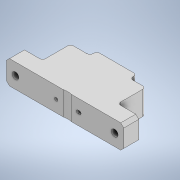
# Autodesk Inventor part: ADAPTER_new-focus-8821
Saved by Autodesk Inventor 2020 (Build 240168000, 168)
## iProperties
Created: 2021-08-06
Part Number: ADAPTER_new-focus-8821
Material: Generic
Document SubType Name: Modeling
Designer: paige
Density: 1 g/cm^3
Appearance: Default
Author: paige
Autodesk Inventor part; units mm, degrees
ref_plane "YZ Plane" through (0, 0, 0) normal (1, 0, 0) x (0, 1, 0)
ref_plane "XZ Plane" through (0, 0, 0) normal (0, 1, 0) x (-1, 0, 0)
ref_plane "XY Plane" through (0, 0, 0) normal (0, 0, 1) x (1, 0, 0)
sketch "Sketch1" plane through (0, 0, 0) normal (0, 0, 1) x (1, 0, 0)
  line L0 (-38.9875, 7.874) -> (38.9875, 7.874)
  line L1 (38.9875, 7.874) -> (38.9875, -7.874)
  line L2 (38.9875, -7.874) -> (-38.9875, -7.874)
  line L3 (-38.9875, -7.874) -> (-38.9875, 7.874)
  point P0 (0, 0)
  dimension "d2" = 77.975
  dimension "d3" = 38.9875
  dimension "d6" = 15.748
  dimension "d7" = 7.874
  constraints: 8 end point, 2 parallel, 1 horizontal, 1 perpendicular
  measures "d2" distance of L0.start L0.end
  measures "d3" distance from line of L1 point (0, 0)
  measures "d6" distance of L2.end L0.start
  measures "d7" distance from line of L2 point (0, 0)
extrude "Extrusion1" add sketch "Sketch1" along normal blind 33.1075
sketch "Sketch2" plane through (0, 0, 0) normal (0, 0, -1) x (-1, 0, 0)
  line L0 (38.9875, 7.874) -> (38.9875, -7.874) projected
  line L1 (-38.9875, -7.874) -> (-38.9875, 7.874) projected
  line L2 (38.9875, -7.874) -> (-38.9875, -7.874) projected
  line L3 (-38.9875, 7.874) -> (38.9875, 7.874) projected
  line L4 (38.9875, -7.874) -> (26.9875, -7.874)
  line L5 (26.9875, -7.874) -> (26.9875, 7.874)
  line L6 (26.9875, 7.874) -> (38.9875, 7.874)
  line L7 (38.9875, 7.874) -> (38.9875, -7.874)
  line L8 (-38.9875, -7.874) -> (-26.9875, -7.874)
  line L9 (-26.9875, -7.874) -> (-26.9875, 7.874)
  line L10 (-26.9875, 7.874) -> (-38.9875, 7.874)
  line L11 (-38.9875, 7.874) -> (-38.9875, -7.874)
  line L12 (38.9875, -7.874) -> (-38.9875, -7.874) projected
  line L13 (12.0525, -7.874) -> (-14.5415, -7.874)
  line L14 (-14.5415, -7.874) -> (-14.5415, 7.874)
  line L15 (-14.5415, 7.874) -> (12.0525, 7.874)
  line L16 (12.0525, 7.874) -> (12.0525, -7.874)
  line L17 (26.9875, -7.874) -> (12.0525, -7.874)
  line L18 (12.0525, -7.874) -> (12.0525, 7.874)
  line L19 (12.0525, 7.874) -> (26.9875, 7.874)
  line L20 (26.9875, 7.874) -> (26.9875, -7.874)
  line L21 (-14.5415, -7.874) -> (-26.9875, -7.874)
  line L22 (-26.9875, -7.874) -> (-26.9875, 7.874)
  line L23 (-26.9875, 7.874) -> (-14.5415, 7.874)
  line L24 (-14.5415, 7.874) -> (-14.5415, -7.874)
  line L25 (26.9875, -7.874) -> (24.9875, -7.874)
  line L26 (24.9875, -7.874) -> (24.9875, 7.874)
  line L27 (24.9875, 7.874) -> (26.9875, 7.874)
  line L28 (26.9875, 7.874) -> (26.9875, -7.874)
  line L29 (-26.9875, -7.874) -> (-24.9875, -7.874)
  line L30 (-24.9875, -7.874) -> (-24.9875, 7.874)
  line L31 (-24.9875, 7.874) -> (-26.9875, 7.874)
  line L32 (-26.9875, 7.874) -> (-26.9875, -7.874)
  point P0 (0, 0)
  point P1 (38.9875, 0)
  point P2 (-38.9875, 0)
  point P3 (-1.5875, 0)
  point P4 (32.9875, 0)
  point P5 (-32.9875, 0)
  point P6 (-14.5415, -7.874)
  point P7 (-24.9875, 7.874)
  point P8 (24.9875, 7.874)
  dimension "d4" = 0
  dimension "d5" = 0
  dimension "d8" = 12
  dimension "d9" = 12
  dimension "d14" = 6
  dimension "d15" = 15.748
  dimension "d16" = 7.874
  dimension "d17" = 6
  dimension "d18" = 7.874
  dimension "d19" = 12.954
  dimension "d20" = 13.64
  dimension "d72" = 25.4
  dimension "d74" = 7.874
  dimension "d83" = 2
  dimension "d84" = 2
  constraints: 56 end point, 14 parallel, 7 horizontal, 7 perpendicular, 6 point on line, 2 midpoint
  measures "d4" vertical distance of point (38.987, 0) point (0, 0)
  measures "d5" vertical distance of point (0, 0) point (-38.987, 0)
  measures "d8" distance between parallel lines of L5 L0
  measures "d9" distance between parallel lines of L1 L9
  measures "d14" distance from line of L5 point (32.987, 0)
  measures "d15" distance of L0.start L0.end
  measures "d16" distance from line of L2 point (32.987, 0)
  measures "d17" distance from line of L9 point (-32.987, 0)
  measures "d18" distance from line of L2 point (-32.987, 0)
  measures "d19" distance from line of L14 point (-1.587, 0)
  measures "d20" distance from line of L16 point (-1.587, 0)
  measures "d72" distance from line of L22 point (-1.587, 0)
  measures "d74" distance from line of L12 point (-1.587, 0)
  measures "d83" distance between parallel lines of L26 L20
  measures "d84" distance between parallel lines of L30 L9
hole "Hole1" at (-32.9875, 0, 0) at (32.9875, 0, 0) direction (0, 0, 1) diameter 4.5 end through all counterbore diameter 8 counterbore depth 30.11 clearance for "Socket Head Cap Screw" size "#8" standard "Ansi Unified Screw Threads"
sketch "Sketch4" plane through (0, 0, 33.1075) normal (0, 0, 1) x (1, 0, 0)
  line L0 (38.9875, 7.874) -> (38.9875, -7.874)
  line L1 (-38.9875, -7.874) -> (-38.9875, 7.874)
  line L2 (38.9875, -7.874) -> (-38.9875, -7.874)
  line L3 (-38.9875, 7.874) -> (38.9875, 7.874)
  line L4 (38.9875, -7.874) -> (26.9875, -7.874)
  line L5 (26.9875, -7.874) -> (26.9875, 7.874)
  line L6 (26.9875, 7.874) -> (38.9875, 7.874)
  line L7 (38.9875, 7.874) -> (38.9875, -7.874)
  line L8 (-38.9875, -7.874) -> (-26.9875, -7.874)
  line L9 (-26.9875, -7.874) -> (-26.9875, 7.874)
  line L10 (-26.9875, 7.874) -> (-38.9875, 7.874)
  line L11 (-38.9875, 7.874) -> (-38.9875, -7.874)
  line L12 (38.9875, -7.874) -> (-38.9875, -7.874)
  line L13 (14.5415, -7.874) -> (-12.0525, -7.874)
  line L14 (-12.0525, -7.874) -> (-12.0525, 7.874)
  line L15 (-12.0525, 7.874) -> (14.5415, 7.874)
  line L16 (14.5415, 7.874) -> (14.5415, -7.874)
  line L17 (26.9875, -7.874) -> (14.5415, -7.874)
  line L18 (14.5415, -7.874) -> (14.5415, 7.874)
  line L19 (14.5415, 7.874) -> (26.9875, 7.874)
  line L20 (26.9875, 7.874) -> (26.9875, -7.874)
  line L21 (-12.0525, -7.874) -> (-26.9875, -7.874)
  line L22 (-26.9875, -7.874) -> (-26.9875, 7.874)
  line L23 (-26.9875, 7.874) -> (-12.0525, 7.874)
  line L24 (-12.0525, 7.874) -> (-12.0525, -7.874)
  point P0 (0, 0)
  point P1 (0, 0)
  point P2 (0, 0)
  point P3 (38.9875, 0)
  point P4 (-38.9875, 0)
  point P5 (1.5875, 0.076)
  point P6 (32.9875, 0)
  point P7 (-32.9875, 0)
  dimension "d48" = 0
  dimension "d49" = 0
  dimension "d50" = 12
  dimension "d51" = 12
  dimension "d54" = 6
  dimension "d55" = 15.748
  dimension "d56" = 7.874
  dimension "d57" = 6
  dimension "d58" = 7.874
  dimension "d59" = 13.64
  dimension "d60" = 12.954
  dimension "d61" = 25.4
  dimension "d75" = 7.95
  constraints: 50 end point, 10 parallel, 5 horizontal, 5 perpendicular, 4 point on line, 2 midpoint
  measures "d48" vertical distance of point (38.987, 0) point (0, 0)
  measures "d49" vertical distance of point (0, 0) point (-38.987, 0)
  measures "d50" distance between parallel lines of L5 L0
  measures "d51" distance between parallel lines of L1 L9
  measures "d54" distance from line of L5 point (32.987, 0)
  measures "d55" distance of L0.start L0.end
  measures "d56" distance from line of L2 point (32.987, 0)
  measures "d57" distance from line of L9 point (-32.987, 0)
  measures "d58" distance from line of L2 point (-32.987, 0)
  measures "d59" distance from line of L14 point (1.587, 0.076)
  measures "d60" distance from line of L16 point (1.587, 0.076)
  measures "d61" distance from line of L5 point (1.587, 0.076)
  measures "d75" distance from line of L2 point (1.587, 0.076)
hole "Hole3" [suppressed]
extrude "Extrusion2" cut sketch "Sketch2" against normal blind 4.508 contours L5 L2 L26 L3 | L26 L2 L16 L3 | L14 L2 L30 L3 | L30 L2 L9 L3
fillet "Fillet1" radius 2 2 edges at (-12.0525, 0, 0) (14.5415, 0, 0)
fillet "Fillet2" radius 2 2 edges at (-12.0525, 0, 4.508) (14.5415, 0, 4.508)
extrude "Extrusion3" cut sketch "Sketch2" against normal blind 23.11 contours L0 L2 L5 L3 | L5 L2 L26 L3 | L30 L2 L9 L3 | L9 L2 L1 L3
chamfer "Chamfer1" distance 2 angle 45 4 edges at (-38.9875, 7.874, 28.1088) (-38.9875, -7.874, 28.1088) (38.9875, 7.874, 28.1088) (38.9875, -7.874, 28.1088)
fillet "Fillet4" radius 2 4 edges at (-24.9875, 0, 4.508) (-24.9875, 0, 23.11) (24.9875, 0, 4.508) (24.9875, 0, 23.11)
sketch "Sketch5" plane through (-10.0525, -7.874, 0) normal (0, -1, 0) x (1, 0, 0)
  line L0 (13.89, 2.9975) -> (9.39, 2.9975) projected
  line L1 (-26.935, 33.1075) -> (47.04, 33.1075) projected
  circle A0 centre (11.64, 45.4575) radius 12.7
  point P0 (10.0525, 0)
  point P1 (11.64, 2.9975)
  point P2 (11.64, 33.1075)
  point P3 (14.601, 33.1075)
  point P4 (8.679, 33.1075)
  dimension "d86" = 25.4
  dimension "d87" = 12.35
  constraints: 1 centre point, 1 midpoint, 1 point on line
  measures "d86" diameter of A0
  measures "d87" distance of A0.centre point (11.64, 33.108)
extrude "Extrusion4" cut sketch "Sketch5" against normal through all contours L1 A0 picked at (11.9717, 33.0038)
sketch "Sketch6" plane through (0, 0, 33.1075) normal (0, 0, 1) x (1, 0, 0)
  line L0 (9.5855, 0) -> (8.5895, 0) construction
  line L1 (9.5855, 1.05) -> (8.5895, 1.05)
  line L2 (8.5895, -1.05) -> (9.5855, -1.05)
  arc A0 (9.5855, -1.05) -> (9.5855, 1.05) centre (9.5855, 0) ccw
  arc A1 (8.5895, 1.05) -> (8.5895, -1.05) centre (8.5895, 0) ccw
  line L3 (-12.0525, 7.874) -> (-12.0525, -7.874) projected
  line L4 (4.5485, -7.874) -> (-1.3735, -7.874) projected
  point P0 (0, 0)
  point P1 (1.5875, -5.5)
  point P2 (1.5875, 0)
  point P3 (-5.9125, 0)
  point P4 (9.0875, 0)
  dimension "d90" = 0
  dimension "d91" = 5.5
  dimension "d92" = 0
  dimension "d93" = 7.5
  dimension "d94" = 0
  dimension "d95" = 7.5
  dimension "d96" = 1.05
  dimension "d97" = 0.996
  dimension "d98" = 13.64
  dimension "d99" = 7.874
  constraints: 8 end point, 4 point on circle, 4 tangent, 2 centre point, 1 horizontal, 1 midpoint, 1 parallel
  measures "d90" horizontal distance of point (1.587, -5.5) point (1.587, 0)
  measures "d91" distance of point (1.587, 0) point (1.587, -5.5)
  measures "d92" vertical distance of point (1.587, 0) point (9.087, 0)
  measures "d93" distance of point (1.587, 0) point (9.087, 0)
  measures "d94" vertical distance of point (1.587, 0) point (-5.913, 0)
  measures "d95" distance of point (1.587, 0) point (-5.913, 0)
  measures "d96" radius of A1
  measures "d97" distance of L0.start L0.end
  measures "d98" distance from line of L3 point (1.587, 0)
  measures "d99" distance from line of L4 point (1.587, 0)
hole "Hole4" at (-5.9125, 0, 33.1075) direction (0, 0, -1) diameter 2.1 depth 2.1
sketch "Sketch8" plane through (0, 0, 33.1075) normal (0, 0, 1) x (1, 0, 0)
  line L0 (9.5855, 0) -> (8.5895, 0) construction
  line L1 (9.5855, 1.05) -> (8.5895, 1.05)
  line L2 (8.5895, -1.05) -> (9.5855, -1.05)
  arc A0 (9.5855, -1.05) -> (9.5855, 1.05) centre (9.5855, 0) ccw
  arc A1 (8.5895, 1.05) -> (8.5895, -1.05) centre (8.5895, 0) ccw
  line L3 (-12.0525, 7.874) -> (-12.0525, -7.874)
  line L4 (4.5485, -7.798) -> (-1.3735, -7.798)
  line L5 (4.5485, -7.874) -> (-1.3735, -7.874) projected
  point P0 (0, 0)
  point P1 (0, 0)
  point P2 (1.5875, -5.5)
  point P3 (1.5875, 0)
  point P4 (-5.9125, 0)
  point P5 (9.0875, 0)
  dimension "d121" = 0
  dimension "d122" = 5.5
  dimension "d123" = 0
  dimension "d124" = 7.5
  dimension "d125" = 0
  dimension "d126" = 7.5
  dimension "d127" = 1.05
  dimension "d128" = 0.996
  dimension "d129" = 13.64
  dimension "d157" = 7.874
  constraints: 12 end point, 4 point on circle, 4 tangent, 2 centre point, 1 horizontal, 1 midpoint, 1 parallel
  measures "d121" horizontal distance of point (1.587, -5.5) point (1.587, 0)
  measures "d122" distance of point (1.587, 0) point (1.587, -5.5)
  measures "d123" vertical distance of point (1.587, 0) point (9.087, 0)
  measures "d124" distance of point (1.587, 0) point (9.087, 0)
  measures "d125" vertical distance of point (1.587, 0) point (-5.913, 0)
  measures "d126" distance of point (1.587, 0) point (-5.913, 0)
  measures "d127" radius of A1
  measures "d128" distance of L0.start L0.end
  measures "d129" distance from line of L3 point (1.587, 0)
  measures "d157" distance from line of L5 point (1.587, 0)
extrude "Extrusion6" cut sketch "Sketch8" against normal blind 2.1
sketch "Sketch9" plane through (0, 0, 0) normal (0, 0, -1) x (-1, 0, 0)
  line L0 (38.9875, 7.874) -> (38.9875, -7.874)
  line L1 (-38.9875, -7.874) -> (-38.9875, 7.874)
  line L2 (38.9875, -7.874) -> (-38.9875, -7.874)
  line L3 (-38.9875, 7.874) -> (38.9875, 7.874)
  line L4 (38.9875, -7.874) -> (26.9875, -7.874)
  line L5 (26.9875, -7.874) -> (26.9875, 7.874)
  line L6 (26.9875, 7.874) -> (38.9875, 7.874)
  line L7 (38.9875, 7.874) -> (38.9875, -7.874)
  line L8 (-38.9875, -7.874) -> (-26.9875, -7.874)
  line L9 (-26.9875, -7.874) -> (-26.9875, 7.874)
  line L10 (-26.9875, 7.874) -> (-38.9875, 7.874)
  line L11 (-38.9875, 7.874) -> (-38.9875, -7.874)
  line L12 (38.9875, -7.874) -> (-38.9875, -7.874)
  line L13 (12.0525, -7.874) -> (-14.5415, -7.874)
  line L14 (-14.5415, -7.874) -> (-14.5415, 7.874)
  line L15 (-14.5415, 7.874) -> (12.0525, 7.874)
  line L16 (12.0525, 7.874) -> (12.0525, -7.874)
  line L17 (26.9875, -7.874) -> (12.0525, -7.874)
  line L18 (12.0525, -7.874) -> (12.0525, 7.874)
  line L19 (12.0525, 7.874) -> (26.9875, 7.874)
  line L20 (26.9875, 7.874) -> (26.9875, -7.874)
  line L21 (-14.5415, -7.874) -> (-26.9875, -7.874)
  line L22 (-26.9875, -7.874) -> (-26.9875, 7.874)
  line L23 (-26.9875, 7.874) -> (-14.5415, 7.874)
  line L24 (-14.5415, 7.874) -> (-14.5415, -7.874)
  line L25 (26.9875, -7.874) -> (24.9875, -7.874)
  line L26 (24.9875, -7.874) -> (24.9875, 7.874)
  line L27 (24.9875, 7.874) -> (26.9875, 7.874)
  line L28 (26.9875, 7.874) -> (26.9875, -7.874)
  line L29 (-26.9875, -7.874) -> (-24.9875, -7.874)
  line L30 (-24.9875, -7.874) -> (-24.9875, 7.874)
  line L31 (-24.9875, 7.874) -> (-26.9875, 7.874)
  line L32 (-26.9875, 7.874) -> (-26.9875, -7.874)
  point P0 (0, 0)
  point P1 (0, 0)
  point P2 (38.9875, 0)
  point P3 (-38.9875, 0)
  point P4 (-1.5875, 0.076)
  point P5 (32.9875, 0)
  point P6 (-32.9875, 0)
  point P7 (-14.5415, -7.874)
  point P8 (-24.9875, 7.874)
  point P9 (24.9875, 7.874)
  dimension "d135" = 0
  dimension "d136" = 0
  dimension "d137" = 12
  dimension "d138" = 12
  dimension "d139" = 6
  dimension "d140" = 15.748
  dimension "d141" = 7.874
  dimension "d142" = 6
  dimension "d143" = 7.874
  dimension "d144" = 12.954
  dimension "d145" = 13.64
  dimension "d146" = 25.4
  dimension "d147" = 7.95
  dimension "d148" = 2
  dimension "d149" = 2
  constraints: 66 end point, 14 parallel, 7 horizontal, 7 perpendicular, 6 point on line, 2 midpoint
  measures "d135" vertical distance of point (38.987, 0) point (0, 0)
  measures "d136" vertical distance of point (0, 0) point (-38.987, 0)
  measures "d137" distance between parallel lines of L5 L0
  measures "d138" distance between parallel lines of L1 L9
  measures "d139" distance from line of L5 point (32.987, 0)
  measures "d140" distance of L0.start L0.end
  measures "d141" distance from line of L2 point (32.987, 0)
  measures "d142" distance from line of L9 point (-32.987, 0)
  measures "d143" distance from line of L2 point (-32.987, 0)
  measures "d144" distance from line of L14 point (-1.587, 0.076)
  measures "d145" distance from line of L16 point (-1.587, 0.076)
  measures "d146" distance from line of L22 point (-1.587, 0.076)
  measures "d147" distance from line of L12 point (-1.587, 0.076)
  measures "d148" distance between parallel lines of L26 L20
  measures "d149" distance between parallel lines of L30 L9
hole "Hole5" at (1.5875, 0.076, 0) direction (0, 0, 1) diameter 3.302 depth 12.3 thread size "8-32 UNC" class "2B" standard "ANSI Unified Screw Threads"
equation "\"d3\" = 0.5 * d2"
equation "\"d7\" = 0.5 * d6"
equation "\"d14\" = 0.5 * d8"
equation "\"d17\" = d14"
equation "\"d18\" = d16"
equation "\"d74\" = d18"
equation "\"d54\" = 0.5 * d50"
equation "\"d56\" = 0.5 * d55"
equation "\"d57\" = d54"
equation "\"d58\" = d56"
equation "\"d95\" = d93"
equation "\"d98\" = d59"
equation "\"d99\" = d16"
equation "\"d126\" = d124"
equation "\"d129\" = d131"
equation "\"d157\" = d16"
equation "\"d139\" = 0.5 * d137"
equation "\"d141\" = 0.5 * d140"
equation "\"d142\" = d139"
equation "\"d143\" = d141"
equation "\"d131\" = 13.64"
body "Solid1"
